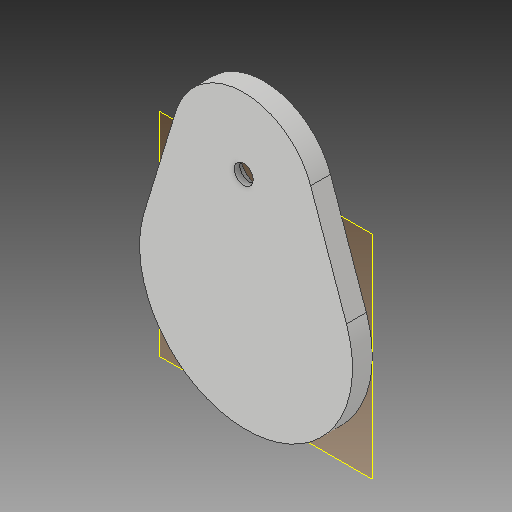
# Autodesk Inventor part: case part 1
Saved by Autodesk Inventor 2017 (Build 210142000, 142)
## iProperties
Created: 2018-04-16
Part Number: case part 1
Material: Generic
Document SubType Name: Modeling
Designer: RKL
Density: 1 g/cm^3
Appearance: Default
Author: RKL
Autodesk Inventor part; units mm, degrees
ref_plane "YZ Plane" through (0, 0, 0) normal (1, 0, 0) x (0, 1, 0)
ref_plane "XZ Plane" through (0, 0, 0) normal (0, 1, 0) x (-1, 0, 0)
ref_plane "XY Plane" through (0, 0, 0) normal (0, 0, 1) x (1, 0, 0)
ref_plane "Work Plane1" through (0, 0, 0) normal (0, 0, 1) x (1, 0, 0)
sketch "Sketch1" plane through (0, 0, 0) normal (0, 0, 1) x (1, 0, 0)
  circle A0 centre (0, 0) radius 17.5 projected
  circle A1 centre (-1.6604, 79.9828) radius 17.5 projected
  circle A2 centre (0, 0) radius 6.7352 construction
  arc A3 (6.3355, 64.3254) -> (5.4562, 67.7807) centre (-13.8587, 61.0262) ccw construction
  arc A4 (5.4562, 67.7807) -> (4.2455, 67.8673) centre (0, 0) ccw construction
  arc A5 (4.2455, 67.8673) -> (2.8834, 64.5723) centre (22.4025, 58.4327) ccw construction
  arc A6 (2.8834, 64.5723) -> (1.7304, 64.6134) centre (0, 0) ccw construction
  arc A7 (1.7304, 64.6134) -> (0.6069, 67.9973) centre (-18.1769, 59.882) ccw construction
  arc A8 (0.6069, 67.9973) -> (-0.6069, 67.9973) centre (0, 0) ccw construction
  arc A9 (-0.6069, 67.9973) -> (-1.7304, 64.6134) centre (18.1769, 59.882) ccw construction
  arc A10 (-1.7304, 64.6134) -> (-2.8834, 64.5723) centre (0, 0) ccw construction
  arc A11 (-2.8834, 64.5723) -> (-4.2455, 67.8673) centre (-22.4025, 58.4327) ccw construction
  arc A12 (-4.2455, 67.8673) -> (-5.4562, 67.7807) centre (0, 0) ccw construction
  arc A13 (-5.4562, 67.7807) -> (-6.3355, 64.3254) centre (13.8587, 61.0262) ccw construction
  arc A14 (-6.3355, 64.3254) -> (-7.4826, 64.202) centre (0, 0) ccw construction
  arc A15 (-7.4826, 64.202) -> (-9.0763, 67.3915) centre (-26.514, 56.6857) ccw construction
  arc A16 (-9.0763, 67.3915) -> (-10.2777, 67.2188) centre (0, 0) ccw construction
  arc A17 (-10.2777, 67.2188) -> (-10.9083, 63.7095) centre (9.4698, 61.8594) ccw construction
  arc A18 (-10.9083, 63.7095) -> (-12.0437, 63.5047) centre (0, 0) ccw construction
  arc A19 (-12.0437, 63.5047) -> (-13.8608, 66.5723) centre (-30.4904, 54.6497) ccw construction
  arc A20 (-13.8608, 66.5723) -> (-15.0469, 66.3143) centre (0, 0) ccw construction
  arc A21 (-15.0469, 66.3143) -> (-15.4255, 62.769) centre (5.0327, 62.3773) ccw construction
  arc A22 (-15.4255, 62.769) -> (-16.5434, 62.4837) centre (0, 0) ccw construction
  arc A23 (-16.5434, 62.4837) -> (-18.5747, 65.4139) centre (-34.3113, 52.3353) ccw construction
  arc A24 (-18.5747, 65.4139) -> (-19.7394, 65.0719) centre (0, 0) ccw construction
  arc A25 (-19.7394, 65.0719) -> (-19.8641, 61.5086) centre (0.5699, 62.5774) ccw construction
  arc A26 (-19.8641, 61.5086) -> (-20.9588, 61.1443) centre (0, 0) ccw construction
  arc A27 (-20.9588, 61.1443) -> (-23.194, 63.9221) centre (-37.9575, 49.7543) ccw construction
  arc A28 (-23.194, 63.9221) -> (-24.3312, 63.498) centre (0, 0) ccw construction
  arc A29 (-24.3312, 63.498) -> (-24.2014, 59.9348) centre (-3.8958, 62.4586) ccw construction
  arc A30 (-24.2014, 59.9348) -> (-25.2673, 59.4933) centre (0, 0) ccw construction
  arc A31 (-25.2673, 59.4933) -> (-27.695, 62.1046) centre (-41.4102, 46.9196) ccw construction
  arc A32 (-27.695, 62.1046) -> (-28.7991, 61.6004) centre (0, 0) ccw construction
  arc A33 (-28.7991, 61.6004) -> (-28.4155, 58.0556) centre (-8.3416, 62.0216) ccw construction
  arc A34 (-28.4155, 58.0556) -> (-29.4472, 57.5392) centre (0, 0) ccw construction
  arc A35 (-29.4472, 57.5392) -> (-32.055, 59.9706) centre (-44.6519, 43.8459) ccw construction
  arc A36 (-32.055, 59.9706) -> (-33.1203, 59.3889) centre (0, 0) ccw construction
  arc A37 (-33.1203, 59.3889) -> (-32.4847, 55.8806) centre (-12.7449, 61.2685) ccw construction
  arc A38 (-32.4847, 55.8806) -> (-33.4769, 55.2918) centre (0, 0) ccw construction
  arc A39 (-33.4769, 55.2918) -> (-36.2516, 57.5311) centre (-47.6661, 40.5488) ccw construction
  arc A40 (-36.2516, 57.5311) -> (-37.2727, 56.8749) centre (0, 0) ccw construction
  arc A41 (-37.2727, 56.8749) -> (-36.3884, 53.4207) centre (-17.0833, 60.2031) ccw construction
  arc A42 (-36.3884, 53.4207) -> (-37.3361, 52.7627) centre (0, 0) ccw construction
  arc A43 (-37.3361, 52.7627) -> (-40.2634, 54.7983) centre (-50.4373, 37.045) ccw construction
  arc A44 (-40.2634, 54.7983) -> (-41.2351, 54.0709) centre (0, 0) ccw construction
  arc A45 (-41.2351, 54.0709) -> (-40.1067, 50.6887) centre (-21.3346, 58.831) ccw construction
  arc A46 (-40.1067, 50.6887) -> (-41.005, 49.9648) centre (0, 0) ccw construction
  arc A47 (-41.005, 49.9648) -> (-44.0701, 51.7864) centre (-52.9516, 33.3525) ccw construction
  arc A48 (-44.0701, 51.7864) -> (-44.9874, 50.9915) centre (0, 0) ccw construction
  arc A49 (-44.9874, 50.9915) -> (-43.6206, 47.6984) centre (-25.4772, 57.1592) ccw construction
  arc A50 (-43.6206, 47.6984) -> (-44.465, 46.9122) centre (0, 0) ccw construction
  arc A51 (-44.465, 46.9122) -> (-47.6522, 48.5105) centre (-55.196, 29.49) ccw construction
  arc A52 (-47.6522, 48.5105) -> (-48.5105, 47.6522) centre (0, 0) ccw construction
  arc A53 (-48.5105, 47.6522) -> (-46.9122, 44.465) centre (-29.49, 55.196) ccw construction
  arc A54 (-46.9122, 44.465) -> (-47.6984, 43.6206) centre (0, 0) ccw construction
  arc A55 (-47.6984, 43.6206) -> (-50.9915, 44.9874) centre (-57.1592, 25.4772) ccw construction
  arc A56 (-50.9915, 44.9874) -> (-51.7864, 44.0701) centre (0, 0) ccw construction
  arc A57 (-51.7864, 44.0701) -> (-49.9648, 41.005) centre (-33.3525, 52.9516) ccw construction
  arc A58 (-49.9648, 41.005) -> (-50.6887, 40.1067) centre (0, 0) ccw construction
  arc A59 (-50.6887, 40.1067) -> (-54.0709, 41.2351) centre (-58.831, 21.3346) ccw construction
  arc A60 (-54.0709, 41.2351) -> (-54.7983, 40.2634) centre (0, 0) ccw construction
  arc A61 (-54.7983, 40.2634) -> (-52.7627, 37.3361) centre (-37.045, 50.4373) ccw construction
  arc A62 (-52.7627, 37.3361) -> (-53.4207, 36.3884) centre (0, 0) ccw construction
  arc A63 (-53.4207, 36.3884) -> (-56.8749, 37.2727) centre (-60.2031, 17.0833) ccw construction
  arc A64 (-56.8749, 37.2727) -> (-57.5311, 36.2516) centre (0, 0) ccw construction
  arc A65 (-57.5311, 36.2516) -> (-55.2918, 33.4769) centre (-40.5488, 47.6661) ccw construction
  arc A66 (-55.2918, 33.4769) -> (-55.8806, 32.4847) centre (0, 0) ccw construction
  arc A67 (-55.8806, 32.4847) -> (-59.3889, 33.1203) centre (-61.2685, 12.7449) ccw construction
  arc A68 (-59.3889, 33.1203) -> (-59.9706, 32.055) centre (0, 0) ccw construction
  arc A69 (-59.9706, 32.055) -> (-57.5392, 29.4472) centre (-43.8459, 44.6519) ccw construction
  arc A70 (-57.5392, 29.4472) -> (-58.0556, 28.4155) centre (0, 0) ccw construction
  arc A71 (-58.0556, 28.4155) -> (-61.6004, 28.7991) centre (-62.0216, 8.3416) ccw construction
  arc A72 (-61.6004, 28.7991) -> (-62.1046, 27.695) centre (0, 0) ccw construction
  arc A73 (-62.1046, 27.695) -> (-59.4933, 25.2673) centre (-46.9196, 41.4102) ccw construction
  arc A74 (-59.4933, 25.2673) -> (-59.9348, 24.2014) centre (0, 0) ccw construction
  arc A75 (-59.9348, 24.2014) -> (-63.498, 24.3312) centre (-62.4586, 3.8958) ccw construction
  arc A76 (-63.498, 24.3312) -> (-63.9221, 23.194) centre (0, 0) ccw construction
  arc A77 (-63.9221, 23.194) -> (-61.1443, 20.9588) centre (-49.7543, 37.9575) ccw construction
  arc A78 (-61.1443, 20.9588) -> (-61.5086, 19.8641) centre (0, 0) ccw construction
  arc A79 (-61.5086, 19.8641) -> (-65.0719, 19.7394) centre (-62.5774, -0.5699) ccw construction
  arc A80 (-65.0719, 19.7394) -> (-65.4139, 18.5747) centre (0, 0) ccw construction
  arc A81 (-65.4139, 18.5747) -> (-62.4837, 16.5434) centre (-52.3353, 34.3113) ccw construction
  arc A82 (-62.4837, 16.5434) -> (-62.769, 15.4255) centre (0, 0) ccw construction
  arc A83 (-62.769, 15.4255) -> (-66.3143, 15.0469) centre (-62.3773, -5.0327) ccw construction
  arc A84 (-66.3143, 15.0469) -> (-66.5723, 13.8608) centre (0, 0) ccw construction
  arc A85 (-66.5723, 13.8608) -> (-63.5047, 12.0437) centre (-54.6497, 30.4904) ccw construction
  arc A86 (-63.5047, 12.0437) -> (-63.7095, 10.9083) centre (0, 0) ccw construction
  arc A87 (-63.7095, 10.9083) -> (-67.2188, 10.2777) centre (-61.8594, -9.4698) ccw construction
  arc A88 (-67.2188, 10.2777) -> (-67.3915, 9.0763) centre (0, 0) ccw construction
  arc A89 (-67.3915, 9.0763) -> (-64.202, 7.4826) centre (-56.6857, 26.514) ccw construction
  arc A90 (-64.202, 7.4826) -> (-64.3254, 6.3355) centre (0, 0) ccw construction
  arc A91 (-64.3254, 6.3355) -> (-67.7807, 5.4562) centre (-61.0262, -13.8587) ccw construction
  arc A92 (-67.7807, 5.4562) -> (-67.8673, 4.2455) centre (0, 0) ccw construction
  arc A93 (-67.8673, 4.2455) -> (-64.5723, 2.8834) centre (-58.4327, 22.4025) ccw construction
  arc A94 (-64.5723, 2.8834) -> (-64.6134, 1.7304) centre (0, 0) ccw construction
  arc A95 (-64.6134, 1.7304) -> (-67.9973, 0.6069) centre (-59.882, -18.1769) ccw construction
  arc A96 (-67.9973, 0.6069) -> (-67.9973, -0.6069) centre (0, 0) ccw construction
  arc A97 (-67.9973, -0.6069) -> (-64.6134, -1.7304) centre (-59.882, 18.1769) ccw construction
  arc A98 (-64.6134, -1.7304) -> (-64.5723, -2.8834) centre (0, 0) ccw construction
  arc A99 (-64.5723, -2.8834) -> (-67.8673, -4.2455) centre (-58.4327, -22.4025) ccw construction
  arc A100 (-67.8673, -4.2455) -> (-67.7807, -5.4562) centre (0, 0) ccw construction
  arc A101 (-67.7807, -5.4562) -> (-64.3254, -6.3355) centre (-61.0262, 13.8587) ccw construction
  arc A102 (-64.3254, -6.3355) -> (-64.202, -7.4826) centre (0, 0) ccw construction
  arc A103 (-64.202, -7.4826) -> (-67.3915, -9.0763) centre (-56.6857, -26.514) ccw construction
  arc A104 (-67.3915, -9.0763) -> (-67.2188, -10.2777) centre (0, 0) ccw construction
  arc A105 (-67.2188, -10.2777) -> (-63.7095, -10.9083) centre (-61.8594, 9.4698) ccw construction
  arc A106 (-63.7095, -10.9083) -> (-63.5047, -12.0437) centre (0, 0) ccw construction
  arc A107 (-63.5047, -12.0437) -> (-66.5723, -13.8608) centre (-54.6497, -30.4904) ccw construction
  arc A108 (-66.5723, -13.8608) -> (-66.3143, -15.0469) centre (0, 0) ccw construction
  arc A109 (-66.3143, -15.0469) -> (-62.769, -15.4255) centre (-62.3773, 5.0327) ccw construction
  arc A110 (-62.769, -15.4255) -> (-62.4837, -16.5434) centre (0, 0) ccw construction
  arc A111 (-62.4837, -16.5434) -> (-65.4139, -18.5747) centre (-52.3353, -34.3113) ccw construction
  arc A112 (-65.4139, -18.5747) -> (-65.0719, -19.7394) centre (0, 0) ccw construction
  arc A113 (-65.0719, -19.7394) -> (-61.5086, -19.8641) centre (-62.5774, 0.5699) ccw construction
  arc A114 (-61.5086, -19.8641) -> (-61.1443, -20.9588) centre (0, 0) ccw construction
  arc A115 (-61.1443, -20.9588) -> (-63.9221, -23.194) centre (-49.7543, -37.9575) ccw construction
  arc A116 (-63.9221, -23.194) -> (-63.498, -24.3312) centre (0, 0) ccw construction
  arc A117 (-63.498, -24.3312) -> (-59.9348, -24.2014) centre (-62.4586, -3.8958) ccw construction
  arc A118 (-59.9348, -24.2014) -> (-59.4933, -25.2673) centre (0, 0) ccw construction
  arc A119 (-59.4933, -25.2673) -> (-62.1046, -27.695) centre (-46.9196, -41.4102) ccw construction
  arc A120 (-62.1046, -27.695) -> (-61.6004, -28.7991) centre (0, 0) ccw construction
  arc A121 (-61.6004, -28.7991) -> (-58.0556, -28.4155) centre (-62.0216, -8.3416) ccw construction
  arc A122 (-58.0556, -28.4155) -> (-57.5392, -29.4472) centre (0, 0) ccw construction
  arc A123 (-57.5392, -29.4472) -> (-59.9706, -32.055) centre (-43.8459, -44.6519) ccw construction
  arc A124 (-59.9706, -32.055) -> (-59.3889, -33.1203) centre (0, 0) ccw construction
  arc A125 (-59.3889, -33.1203) -> (-55.8806, -32.4847) centre (-61.2685, -12.7449) ccw construction
  arc A126 (-55.8806, -32.4847) -> (-55.2918, -33.4769) centre (0, 0) ccw construction
  arc A127 (-55.2918, -33.4769) -> (-57.5311, -36.2516) centre (-40.5488, -47.6661) ccw construction
  arc A128 (-57.5311, -36.2516) -> (-56.8749, -37.2727) centre (0, 0) ccw construction
  arc A129 (-56.8749, -37.2727) -> (-53.4207, -36.3884) centre (-60.2031, -17.0833) ccw construction
  arc A130 (-53.4207, -36.3884) -> (-52.7627, -37.3361) centre (0, 0) ccw construction
  arc A131 (-52.7627, -37.3361) -> (-54.7983, -40.2634) centre (-37.045, -50.4373) ccw construction
  arc A132 (-54.7983, -40.2634) -> (-54.0709, -41.2351) centre (0, 0) ccw construction
  arc A133 (-54.0709, -41.2351) -> (-50.6887, -40.1067) centre (-58.831, -21.3346) ccw construction
  arc A134 (-50.6887, -40.1067) -> (-49.9648, -41.005) centre (0, 0) ccw construction
  arc A135 (-49.9648, -41.005) -> (-51.7864, -44.0701) centre (-33.3525, -52.9516) ccw construction
  arc A136 (-51.7864, -44.0701) -> (-50.9915, -44.9874) centre (0, 0) ccw construction
  arc A137 (-50.9915, -44.9874) -> (-47.6984, -43.6206) centre (-57.1592, -25.4772) ccw construction
  arc A138 (-47.6984, -43.6206) -> (-46.9122, -44.465) centre (0, 0) ccw construction
  arc A139 (-46.9122, -44.465) -> (-48.5105, -47.6522) centre (-29.49, -55.196) ccw construction
  arc A140 (-48.5105, -47.6522) -> (-47.6522, -48.5105) centre (0, 0) ccw construction
  arc A141 (-47.6522, -48.5105) -> (-44.465, -46.9122) centre (-55.196, -29.49) ccw construction
  arc A142 (-44.465, -46.9122) -> (-43.6206, -47.6984) centre (0, 0) ccw construction
  arc A143 (-43.6206, -47.6984) -> (-44.9874, -50.9915) centre (-25.4772, -57.1592) ccw construction
  arc A144 (-44.9874, -50.9915) -> (-44.0701, -51.7864) centre (0, 0) ccw construction
  arc A145 (-44.0701, -51.7864) -> (-41.005, -49.9648) centre (-52.9516, -33.3525) ccw construction
  arc A146 (-41.005, -49.9648) -> (-40.1067, -50.6887) centre (0, 0) ccw construction
  arc A147 (-40.1067, -50.6887) -> (-41.2351, -54.0709) centre (-21.3346, -58.831) ccw construction
  arc A148 (-41.2351, -54.0709) -> (-40.2634, -54.7983) centre (0, 0) ccw construction
  arc A149 (-40.2634, -54.7983) -> (-37.3361, -52.7627) centre (-50.4373, -37.045) ccw construction
  arc A150 (-37.3361, -52.7627) -> (-36.3884, -53.4207) centre (0, 0) ccw construction
  arc A151 (-36.3884, -53.4207) -> (-37.2727, -56.8749) centre (-17.0833, -60.2031) ccw construction
  arc A152 (-37.2727, -56.8749) -> (-36.2516, -57.5311) centre (0, 0) ccw construction
  arc A153 (-36.2516, -57.5311) -> (-33.4769, -55.2918) centre (-47.6661, -40.5488) ccw construction
  arc A154 (-33.4769, -55.2918) -> (-32.4847, -55.8806) centre (0, 0) ccw construction
  arc A155 (-32.4847, -55.8806) -> (-33.1203, -59.3889) centre (-12.7449, -61.2685) ccw construction
  arc A156 (-33.1203, -59.3889) -> (-32.055, -59.9706) centre (0, 0) ccw construction
  arc A157 (-32.055, -59.9706) -> (-29.4472, -57.5392) centre (-44.6519, -43.8459) ccw construction
  arc A158 (-29.4472, -57.5392) -> (-28.4155, -58.0556) centre (0, 0) ccw construction
  arc A159 (-28.4155, -58.0556) -> (-28.7991, -61.6004) centre (-8.3416, -62.0216) ccw construction
  arc A160 (-28.7991, -61.6004) -> (-27.695, -62.1046) centre (0, 0) ccw construction
  arc A161 (-27.695, -62.1046) -> (-25.2673, -59.4933) centre (-41.4102, -46.9196) ccw construction
  arc A162 (-25.2673, -59.4933) -> (-24.2014, -59.9348) centre (0, 0) ccw construction
  arc A163 (-24.2014, -59.9348) -> (-24.3312, -63.498) centre (-3.8958, -62.4586) ccw construction
  arc A164 (-24.3312, -63.498) -> (-23.194, -63.9221) centre (0, 0) ccw construction
  arc A165 (-23.194, -63.9221) -> (-20.9588, -61.1443) centre (-37.9575, -49.7543) ccw construction
  arc A166 (-20.9588, -61.1443) -> (-19.8641, -61.5086) centre (0, 0) ccw construction
  arc A167 (-19.8641, -61.5086) -> (-19.7394, -65.0719) centre (0.5699, -62.5774) ccw construction
  arc A168 (-19.7394, -65.0719) -> (-18.5747, -65.4139) centre (0, 0) ccw construction
  arc A169 (-18.5747, -65.4139) -> (-16.5434, -62.4837) centre (-34.3113, -52.3353) ccw construction
  arc A170 (-16.5434, -62.4837) -> (-15.4255, -62.769) centre (0, 0) ccw construction
  arc A171 (-15.4255, -62.769) -> (-15.0469, -66.3143) centre (5.0327, -62.3773) ccw construction
  arc A172 (-15.0469, -66.3143) -> (-13.8608, -66.5723) centre (0, 0) ccw construction
  arc A173 (-13.8608, -66.5723) -> (-12.0437, -63.5047) centre (-30.4904, -54.6497) ccw construction
  arc A174 (-12.0437, -63.5047) -> (-10.9083, -63.7095) centre (0, 0) ccw construction
  arc A175 (-10.9083, -63.7095) -> (-10.2777, -67.2188) centre (9.4698, -61.8594) ccw construction
  arc A176 (-10.2777, -67.2188) -> (-9.0763, -67.3915) centre (0, 0) ccw construction
  arc A177 (-9.0763, -67.3915) -> (-7.4826, -64.202) centre (-26.514, -56.6857) ccw construction
  arc A178 (-7.4826, -64.202) -> (-6.3355, -64.3254) centre (0, 0) ccw construction
  arc A179 (-6.3355, -64.3254) -> (-5.4562, -67.7807) centre (13.8587, -61.0262) ccw construction
  arc A180 (-5.4562, -67.7807) -> (-4.2455, -67.8673) centre (0, 0) ccw construction
  arc A181 (-4.2455, -67.8673) -> (-2.8834, -64.5723) centre (-22.4025, -58.4327) ccw construction
  arc A182 (-2.8834, -64.5723) -> (-1.7304, -64.6134) centre (0, 0) ccw construction
  arc A183 (-1.7304, -64.6134) -> (-0.6069, -67.9973) centre (18.1769, -59.882) ccw construction
  arc A184 (-0.6069, -67.9973) -> (0.6069, -67.9973) centre (0, 0) ccw construction
  arc A185 (0.6069, -67.9973) -> (1.7304, -64.6134) centre (-18.1769, -59.882) ccw construction
  arc A186 (1.7304, -64.6134) -> (2.8834, -64.5723) centre (0, 0) ccw construction
  arc A187 (2.8834, -64.5723) -> (4.2455, -67.8673) centre (22.4025, -58.4327) ccw construction
  arc A188 (4.2455, -67.8673) -> (5.4562, -67.7807) centre (0, 0) ccw construction
  arc A189 (5.4562, -67.7807) -> (6.3355, -64.3254) centre (-13.8587, -61.0262) ccw construction
  arc A190 (6.3355, -64.3254) -> (7.4826, -64.202) centre (0, 0) ccw construction
  arc A191 (7.4826, -64.202) -> (9.0763, -67.3915) centre (26.514, -56.6857) ccw construction
  arc A192 (9.0763, -67.3915) -> (10.2777, -67.2188) centre (0, 0) ccw construction
  arc A193 (10.2777, -67.2188) -> (10.9083, -63.7095) centre (-9.4698, -61.8594) ccw construction
  arc A194 (10.9083, -63.7095) -> (12.0437, -63.5047) centre (0, 0) ccw construction
  arc A195 (12.0437, -63.5047) -> (13.8608, -66.5723) centre (30.4904, -54.6497) ccw construction
  arc A196 (13.8608, -66.5723) -> (15.0469, -66.3143) centre (0, 0) ccw construction
  arc A197 (15.0469, -66.3143) -> (15.4255, -62.769) centre (-5.0327, -62.3773) ccw construction
  arc A198 (15.4255, -62.769) -> (16.5434, -62.4837) centre (0, 0) ccw construction
  arc A199 (16.5434, -62.4837) -> (18.5747, -65.4139) centre (34.3113, -52.3353) ccw construction
  arc A200 (18.5747, -65.4139) -> (19.7394, -65.0719) centre (0, 0) ccw construction
  arc A201 (19.7394, -65.0719) -> (19.8641, -61.5086) centre (-0.5699, -62.5774) ccw construction
  arc A202 (19.8641, -61.5086) -> (20.9588, -61.1443) centre (0, 0) ccw construction
  arc A203 (20.9588, -61.1443) -> (23.194, -63.9221) centre (37.9575, -49.7543) ccw construction
  arc A204 (23.194, -63.9221) -> (24.3312, -63.498) centre (0, 0) ccw construction
  arc A205 (24.3312, -63.498) -> (24.2014, -59.9348) centre (3.8958, -62.4586) ccw construction
  arc A206 (24.2014, -59.9348) -> (25.2673, -59.4933) centre (0, 0) ccw construction
  arc A207 (25.2673, -59.4933) -> (27.695, -62.1046) centre (41.4102, -46.9196) ccw construction
  arc A208 (27.695, -62.1046) -> (28.7991, -61.6004) centre (0, 0) ccw construction
  arc A209 (28.7991, -61.6004) -> (28.4155, -58.0556) centre (8.3416, -62.0216) ccw construction
  arc A210 (28.4155, -58.0556) -> (29.4472, -57.5392) centre (0, 0) ccw construction
  arc A211 (29.4472, -57.5392) -> (32.055, -59.9706) centre (44.6519, -43.8459) ccw construction
  arc A212 (32.055, -59.9706) -> (33.1203, -59.3889) centre (0, 0) ccw construction
  arc A213 (33.1203, -59.3889) -> (32.4847, -55.8806) centre (12.7449, -61.2685) ccw construction
  arc A214 (32.4847, -55.8806) -> (33.4769, -55.2918) centre (0, 0) ccw construction
  arc A215 (33.4769, -55.2918) -> (36.2516, -57.5311) centre (47.6661, -40.5488) ccw construction
  arc A216 (36.2516, -57.5311) -> (37.2727, -56.8749) centre (0, 0) ccw construction
  arc A217 (37.2727, -56.8749) -> (36.3884, -53.4207) centre (17.0833, -60.2031) ccw construction
  arc A218 (36.3884, -53.4207) -> (37.3361, -52.7627) centre (0, 0) ccw construction
  arc A219 (37.3361, -52.7627) -> (40.2634, -54.7983) centre (50.4373, -37.045) ccw construction
  arc A220 (40.2634, -54.7983) -> (41.2351, -54.0709) centre (0, 0) ccw construction
  arc A221 (41.2351, -54.0709) -> (40.1067, -50.6887) centre (21.3346, -58.831) ccw construction
  arc A222 (40.1067, -50.6887) -> (41.005, -49.9648) centre (0, 0) ccw construction
  arc A223 (41.005, -49.9648) -> (44.0701, -51.7864) centre (52.9516, -33.3525) ccw construction
  arc A224 (44.0701, -51.7864) -> (44.9874, -50.9915) centre (0, 0) ccw construction
  arc A225 (44.9874, -50.9915) -> (43.6206, -47.6984) centre (25.4772, -57.1592) ccw construction
  arc A226 (43.6206, -47.6984) -> (44.465, -46.9122) centre (0, 0) ccw construction
  arc A227 (44.465, -46.9122) -> (47.6522, -48.5105) centre (55.196, -29.49) ccw construction
  arc A228 (47.6522, -48.5105) -> (48.5105, -47.6522) centre (0, 0) ccw construction
  arc A229 (48.5105, -47.6522) -> (46.9122, -44.465) centre (29.49, -55.196) ccw construction
  arc A230 (46.9122, -44.465) -> (47.6984, -43.6206) centre (0, 0) ccw construction
  arc A231 (47.6984, -43.6206) -> (50.9915, -44.9874) centre (57.1592, -25.4772) ccw construction
  arc A232 (50.9915, -44.9874) -> (51.7864, -44.0701) centre (0, 0) ccw construction
  arc A233 (51.7864, -44.0701) -> (49.9648, -41.005) centre (33.3525, -52.9516) ccw construction
  arc A234 (49.9648, -41.005) -> (50.6887, -40.1067) centre (0, 0) ccw construction
  arc A235 (50.6887, -40.1067) -> (54.0709, -41.2351) centre (58.831, -21.3346) ccw construction
  arc A236 (54.0709, -41.2351) -> (54.7983, -40.2634) centre (0, 0) ccw construction
  arc A237 (54.7983, -40.2634) -> (52.7627, -37.3361) centre (37.045, -50.4373) ccw construction
  arc A238 (52.7627, -37.3361) -> (53.4207, -36.3884) centre (0, 0) ccw construction
  arc A239 (53.4207, -36.3884) -> (56.8749, -37.2727) centre (60.2031, -17.0833) ccw construction
  arc A240 (56.8749, -37.2727) -> (57.5311, -36.2516) centre (0, 0) ccw construction
  arc A241 (57.5311, -36.2516) -> (55.2918, -33.4769) centre (40.5488, -47.6661) ccw construction
  arc A242 (55.2918, -33.4769) -> (55.8806, -32.4847) centre (0, 0) ccw construction
  arc A243 (55.8806, -32.4847) -> (59.3889, -33.1203) centre (61.2685, -12.7449) ccw construction
  arc A244 (59.3889, -33.1203) -> (59.9706, -32.055) centre (0, 0) ccw construction
  arc A245 (59.9706, -32.055) -> (57.5392, -29.4472) centre (43.8459, -44.6519) ccw construction
  arc A246 (57.5392, -29.4472) -> (58.0556, -28.4155) centre (0, 0) ccw construction
  arc A247 (58.0556, -28.4155) -> (61.6004, -28.7991) centre (62.0216, -8.3416) ccw construction
  arc A248 (61.6004, -28.7991) -> (62.1046, -27.695) centre (0, 0) ccw construction
  arc A249 (62.1046, -27.695) -> (59.4933, -25.2673) centre (46.9196, -41.4102) ccw construction
  arc A250 (59.4933, -25.2673) -> (59.9348, -24.2014) centre (0, 0) ccw construction
  arc A251 (59.9348, -24.2014) -> (63.498, -24.3312) centre (62.4586, -3.8958) ccw construction
  arc A252 (63.498, -24.3312) -> (63.9221, -23.194) centre (0, 0) ccw construction
  arc A253 (63.9221, -23.194) -> (61.1443, -20.9588) centre (49.7543, -37.9575) ccw construction
  arc A254 (61.1443, -20.9588) -> (61.5086, -19.8641) centre (0, 0) ccw construction
  arc A255 (61.5086, -19.8641) -> (65.0719, -19.7394) centre (62.5774, 0.5699) ccw construction
  arc A256 (65.0719, -19.7394) -> (65.4139, -18.5747) centre (0, 0) ccw construction
  arc A257 (65.4139, -18.5747) -> (62.4837, -16.5434) centre (52.3353, -34.3113) ccw construction
  arc A258 (62.4837, -16.5434) -> (62.769, -15.4255) centre (0, 0) ccw construction
  arc A259 (62.769, -15.4255) -> (66.3143, -15.0469) centre (62.3773, 5.0327) ccw construction
  arc A260 (66.3143, -15.0469) -> (66.5723, -13.8608) centre (0, 0) ccw construction
  arc A261 (66.5723, -13.8608) -> (63.5047, -12.0437) centre (54.6497, -30.4904) ccw construction
  arc A262 (63.5047, -12.0437) -> (63.7095, -10.9083) centre (0, 0) ccw construction
  arc A263 (63.7095, -10.9083) -> (67.2188, -10.2777) centre (61.8594, 9.4698) ccw construction
  arc A264 (67.2188, -10.2777) -> (67.3915, -9.0763) centre (0, 0) ccw construction
  arc A265 (67.3915, -9.0763) -> (64.202, -7.4826) centre (56.6857, -26.514) ccw construction
  arc A266 (64.202, -7.4826) -> (64.3254, -6.3355) centre (0, 0) ccw construction
  arc A267 (64.3254, -6.3355) -> (67.7807, -5.4562) centre (61.0262, 13.8587) ccw construction
  arc A268 (67.7807, -5.4562) -> (67.8673, -4.2455) centre (0, 0) ccw construction
  arc A269 (67.8673, -4.2455) -> (64.5723, -2.8834) centre (58.4327, -22.4025) ccw construction
  arc A270 (64.5723, -2.8834) -> (64.6134, -1.7304) centre (0, 0) ccw construction
  arc A271 (64.6134, -1.7304) -> (67.9973, -0.6069) centre (59.882, 18.1769) ccw construction
  arc A272 (67.9973, -0.6069) -> (67.9973, 0.6069) centre (0, 0) ccw construction
  arc A273 (67.9973, 0.6069) -> (64.6134, 1.7304) centre (59.882, -18.1769) ccw construction
  arc A274 (64.6134, 1.7304) -> (64.5723, 2.8834) centre (0, 0) ccw construction
  arc A275 (64.5723, 2.8834) -> (67.8673, 4.2455) centre (58.4327, 22.4025) ccw construction
  arc A276 (67.8673, 4.2455) -> (67.7807, 5.4562) centre (0, 0) ccw construction
  arc A277 (67.7807, 5.4562) -> (64.3254, 6.3355) centre (61.0262, -13.8587) ccw construction
  arc A278 (64.3254, 6.3355) -> (64.202, 7.4826) centre (0, 0) ccw construction
  arc A279 (64.202, 7.4826) -> (67.3915, 9.0763) centre (56.6857, 26.514) ccw construction
  arc A280 (67.3915, 9.0763) -> (67.2188, 10.2777) centre (0, 0) ccw construction
  arc A281 (67.2188, 10.2777) -> (63.7095, 10.9083) centre (61.8594, -9.4698) ccw construction
  arc A282 (63.7095, 10.9083) -> (63.5047, 12.0437) centre (0, 0) ccw construction
  arc A283 (63.5047, 12.0437) -> (66.5723, 13.8608) centre (54.6497, 30.4904) ccw construction
  arc A284 (66.5723, 13.8608) -> (66.3143, 15.0469) centre (0, 0) ccw construction
  arc A285 (66.3143, 15.0469) -> (62.769, 15.4255) centre (62.3773, -5.0327) ccw construction
  arc A286 (62.769, 15.4255) -> (62.4837, 16.5434) centre (0, 0) ccw construction
  arc A287 (62.4837, 16.5434) -> (65.4139, 18.5747) centre (52.3353, 34.3113) ccw construction
  arc A288 (65.4139, 18.5747) -> (65.0719, 19.7394) centre (0, 0) ccw construction
  arc A289 (65.0719, 19.7394) -> (61.5086, 19.8641) centre (62.5774, -0.5699) ccw construction
  arc A290 (61.5086, 19.8641) -> (61.1443, 20.9588) centre (0, 0) ccw construction
  arc A291 (61.1443, 20.9588) -> (63.9221, 23.194) centre (49.7543, 37.9575) ccw construction
  arc A292 (63.9221, 23.194) -> (63.498, 24.3312) centre (0, 0) ccw construction
  arc A293 (63.498, 24.3312) -> (59.9348, 24.2014) centre (62.4586, 3.8958) ccw construction
  arc A294 (59.9348, 24.2014) -> (59.4933, 25.2673) centre (0, 0) ccw construction
  arc A295 (59.4933, 25.2673) -> (62.1046, 27.695) centre (46.9196, 41.4102) ccw construction
  arc A296 (62.1046, 27.695) -> (61.6004, 28.7991) centre (0, 0) ccw construction
  arc A297 (61.6004, 28.7991) -> (58.0556, 28.4155) centre (62.0216, 8.3416) ccw construction
  arc A298 (58.0556, 28.4155) -> (57.5392, 29.4472) centre (0, 0) ccw construction
  arc A299 (57.5392, 29.4472) -> (59.9706, 32.055) centre (43.8459, 44.6519) ccw construction
  arc A300 (59.9706, 32.055) -> (59.3889, 33.1203) centre (0, 0) ccw construction
  arc A301 (59.3889, 33.1203) -> (55.8806, 32.4847) centre (61.2685, 12.7449) ccw construction
  arc A302 (55.8806, 32.4847) -> (55.2918, 33.4769) centre (0, 0) ccw construction
  arc A303 (55.2918, 33.4769) -> (57.5311, 36.2516) centre (40.5488, 47.6661) ccw construction
  arc A304 (57.5311, 36.2516) -> (56.8749, 37.2727) centre (0, 0) ccw construction
  arc A305 (56.8749, 37.2727) -> (53.4207, 36.3884) centre (60.2031, 17.0833) ccw construction
  arc A306 (53.4207, 36.3884) -> (52.7627, 37.3361) centre (0, 0) ccw construction
  arc A307 (52.7627, 37.3361) -> (54.7983, 40.2634) centre (37.045, 50.4373) ccw construction
  arc A308 (54.7983, 40.2634) -> (54.0709, 41.2351) centre (0, 0) ccw construction
  arc A309 (54.0709, 41.2351) -> (50.6887, 40.1067) centre (58.831, 21.3346) ccw construction
  arc A310 (50.6887, 40.1067) -> (49.9648, 41.005) centre (0, 0) ccw construction
  arc A311 (49.9648, 41.005) -> (51.7864, 44.0701) centre (33.3525, 52.9516) ccw construction
  arc A312 (51.7864, 44.0701) -> (50.9915, 44.9874) centre (0, 0) ccw construction
  arc A313 (50.9915, 44.9874) -> (47.6984, 43.6206) centre (57.1592, 25.4772) ccw construction
  arc A314 (47.6984, 43.6206) -> (46.9122, 44.465) centre (0, 0) ccw construction
  arc A315 (46.9122, 44.465) -> (48.5105, 47.6522) centre (29.49, 55.196) ccw construction
  arc A316 (48.5105, 47.6522) -> (47.6522, 48.5105) centre (0, 0) ccw construction
  arc A317 (47.6522, 48.5105) -> (44.465, 46.9122) centre (55.196, 29.49) ccw construction
  arc A318 (44.465, 46.9122) -> (43.6206, 47.6984) centre (0, 0) ccw construction
  arc A319 (43.6206, 47.6984) -> (44.9874, 50.9915) centre (25.4772, 57.1592) ccw construction
  arc A320 (44.9874, 50.9915) -> (44.0701, 51.7864) centre (0, 0) ccw construction
  arc A321 (44.0701, 51.7864) -> (41.005, 49.9648) centre (52.9516, 33.3525) ccw construction
  arc A322 (41.005, 49.9648) -> (40.1067, 50.6887) centre (0, 0) ccw construction
  arc A323 (40.1067, 50.6887) -> (41.2351, 54.0709) centre (21.3346, 58.831) ccw construction
  arc A324 (41.2351, 54.0709) -> (40.2634, 54.7983) centre (0, 0) ccw construction
  arc A325 (40.2634, 54.7983) -> (37.3361, 52.7627) centre (50.4373, 37.045) ccw construction
  arc A326 (37.3361, 52.7627) -> (36.3884, 53.4207) centre (0, 0) ccw construction
  arc A327 (36.3884, 53.4207) -> (37.2727, 56.8749) centre (17.0833, 60.2031) ccw construction
  arc A328 (37.2727, 56.8749) -> (36.2516, 57.5311) centre (0, 0) ccw construction
  arc A329 (36.2516, 57.5311) -> (33.4769, 55.2918) centre (47.6661, 40.5488) ccw construction
  arc A330 (33.4769, 55.2918) -> (32.4847, 55.8806) centre (0, 0) ccw construction
  arc A331 (32.4847, 55.8806) -> (33.1203, 59.3889) centre (12.7449, 61.2685) ccw construction
  arc A332 (33.1203, 59.3889) -> (32.055, 59.9706) centre (0, 0) ccw construction
  arc A333 (32.055, 59.9706) -> (29.4472, 57.5392) centre (44.6519, 43.8459) ccw construction
  arc A334 (29.4472, 57.5392) -> (28.4155, 58.0556) centre (0, 0) ccw construction
  arc A335 (28.4155, 58.0556) -> (28.7991, 61.6004) centre (8.3416, 62.0216) ccw construction
  arc A336 (28.7991, 61.6004) -> (27.695, 62.1046) centre (0, 0) ccw construction
  arc A337 (27.695, 62.1046) -> (25.2673, 59.4933) centre (41.4102, 46.9196) ccw construction
  arc A338 (25.2673, 59.4933) -> (24.2014, 59.9348) centre (0, 0) ccw construction
  arc A339 (24.2014, 59.9348) -> (24.3312, 63.498) centre (3.8958, 62.4586) ccw construction
  arc A340 (24.3312, 63.498) -> (23.194, 63.9221) centre (0, 0) ccw construction
  arc A341 (23.194, 63.9221) -> (20.9588, 61.1443) centre (37.9575, 49.7543) ccw construction
  arc A342 (20.9588, 61.1443) -> (19.8641, 61.5086) centre (0, 0) ccw construction
  arc A343 (19.8641, 61.5086) -> (19.7394, 65.0719) centre (-0.5699, 62.5774) ccw construction
  arc A344 (19.7394, 65.0719) -> (18.5747, 65.4139) centre (0, 0) ccw construction
  arc A345 (18.5747, 65.4139) -> (16.5434, 62.4837) centre (34.3113, 52.3353) ccw construction
  arc A346 (16.5434, 62.4837) -> (15.4255, 62.769) centre (0, 0) ccw construction
  arc A347 (15.4255, 62.769) -> (15.0469, 66.3143) centre (-5.0327, 62.3773) ccw construction
  arc A348 (15.0469, 66.3143) -> (13.8608, 66.5723) centre (0, 0) ccw construction
  arc A349 (13.8608, 66.5723) -> (12.0437, 63.5047) centre (30.4904, 54.6497) ccw construction
  arc A350 (12.0437, 63.5047) -> (10.9083, 63.7095) centre (0, 0) ccw construction
  arc A351 (10.9083, 63.7095) -> (10.2777, 67.2188) centre (-9.4698, 61.8594) ccw construction
  arc A352 (10.2777, 67.2188) -> (9.0763, 67.3915) centre (0, 0) ccw construction
  arc A353 (9.0763, 67.3915) -> (7.4826, 64.202) centre (26.514, 56.6857) ccw construction
  arc A354 (7.4826, 64.202) -> (6.3355, 64.3254) centre (0, 0) ccw construction
  line L0 (1.5013, 85.9298) -> (4.2866, 76.8211) construction
  line L1 (4.2866, 76.8211) -> (-4.822, 74.0358) construction
  line L2 (-4.822, 74.0358) -> (-7.6074, 83.1444) construction
  line L3 (-7.6074, 83.1444) -> (1.5013, 85.9298) construction
  arc A355 (-2.5253, 42.7312) -> (-0.1223, 36.0097) centre (25.3334, 48.9006) ccw construction
  arc A356 (-0.1223, 36.0097) -> (2.4319, 36.1735) centre (-1.6604, 79.9828) ccw construction
  arc A357 (2.4319, 36.1735) -> (3.9565, 43.1469) centre (-24.462, 45.7067) ccw construction
  arc A358 (3.9565, 43.1469) -> (6.0888, 43.5359) centre (-1.6604, 79.9828) ccw construction
  arc A359 (6.0888, 43.5359) -> (9.9772, 37.5497) centre (31.7738, 55.9636) ccw construction
  arc A360 (9.9772, 37.5497) -> (12.4247, 38.2981) centre (-1.6604, 79.9828) ccw construction
  arc A361 (12.4247, 38.2981) -> (12.3001, 45.4352) centre (-15.9428, 41.3722) ccw construction
  arc A362 (12.3001, 45.4352) -> (14.2852, 46.3054) centre (-1.6604, 79.9828) ccw construction
  arc A363 (14.2852, 46.3054) -> (19.4492, 41.3773) centre (36.4118, 64.3215) ccw construction
  arc A364 (19.4492, 41.3773) -> (21.6582, 42.67) centre (-1.6604, 79.9828) ccw construction
  arc A365 (21.6582, 42.67) -> (19.891, 49.5859) centre (-6.6536, 39.1192) ccw construction
  arc A366 (19.891, 49.5859) -> (21.6219, 50.8905) centre (-1.6604, 79.9828) ccw construction
  arc A367 (21.6219, 50.8905) -> (27.7833, 47.2861) centre (38.9973, 73.5237) ccw construction
  arc A368 (27.7833, 47.2861) -> (29.6346, 49.0534) centre (-1.6604, 79.9828) ccw construction
  arc A369 (29.6346, 49.0534) -> (26.32, 55.3754) centre (2.9048, 39.0691) ccw construction
  arc A370 (26.32, 55.3754) -> (27.7035, 57.0439) centre (-1.6604, 79.9828) ccw construction
  arc A371 (27.7035, 57.0439) -> (34.53, 54.9576) centre (39.3909, 83.0741) ccw construction
  arc A372 (34.53, 54.9576) -> (35.9238, 57.1042) centre (-1.6604, 79.9828) ccw construction
  arc A373 (35.9238, 57.1042) -> (31.2407, 62.4914) centre (12.2171, 41.2248) ccw construction
  arc A374 (31.2407, 62.4914) -> (32.2021, 64.434) centre (-1.6604, 79.9828) ccw construction
  arc A375 (32.2021, 64.434) -> (39.3257, 63.9782) centre (37.5715, 92.4579) ccw construction
  arc A376 (39.3257, 63.9782) -> (40.1869, 66.3884) centre (-1.6604, 79.9828) ccw construction
  arc A377 (40.1869, 66.3884) -> (34.3876, 70.5504) centre (20.7812, 45.4698) ccw construction
  arc A378 (34.3876, 70.5504) -> (34.8751, 72.6623) centre (-1.6604, 79.9828) ccw construction
  arc A379 (34.8751, 72.6623) -> (41.9118, 73.8617) centre (33.637, 101.1691) ccw construction
  arc A380 (41.9118, 73.8617) -> (42.194, 76.4055) centre (-1.6604, 79.9828) ccw construction
  arc A381 (42.194, 76.4055) -> (35.5912, 79.1179) centre (28.1355, 51.5755) ccw construction
  arc A382 (35.5912, 79.1179) -> (35.5785, 81.2853) centre (-1.6604, 79.9828) ccw construction
  arc A383 (35.5785, 81.2853) -> (42.1489, 84.0751) centre (27.7997, 108.7382) ccw construction
  arc A384 (42.1489, 84.0751) -> (41.8368, 86.6154) centre (-1.6604, 79.9828) ccw construction
  arc A385 (41.8368, 86.6154) -> (34.7865, 87.732) centre (33.8835, 59.2126) ccw construction
  arc A386 (34.7865, 87.732) -> (34.2743, 89.8381) centre (-1.6604, 79.9828) ccw construction
  arc A387 (34.2743, 89.8381) -> (40.0243, 94.0679) centre (20.3741, 114.757) ccw construction
  arc A388 (40.0243, 94.0679) -> (39.1348, 96.4678) centre (-1.6604, 79.9828) ccw construction
  arc A389 (39.1348, 96.4678) -> (32.017, 95.9283) centre (37.7154, 67.9695) ccw construction
  arc A390 (32.017, 95.9283) -> (31.0329, 97.8595) centre (-1.6604, 79.9828) ccw construction
  arc A391 (31.0329, 97.8595) -> (35.6524, 103.3014) centre (11.7607, 118.9012) ccw construction
  arc A392 (35.6524, 103.3014) -> (34.2334, 105.4314) centre (-1.6604, 79.9828) ccw construction
  arc A393 (34.2334, 105.4314) -> (27.4319, 103.2651) centre (39.4244, 77.374) ccw construction
  arc A394 (27.4319, 103.2651) -> (26.029, 104.9172) centre (-1.6604, 79.9828) ccw construction
  arc A395 (26.029, 104.9172) -> (29.269, 111.2777) centre (2.4237, 120.9472) ccw construction
  arc A396 (29.269, 111.2777) -> (27.397, 113.0232) centre (-1.6604, 79.9828) ccw construction
  arc A397 (27.397, 113.0232) -> (21.2785, 109.3466) centre (38.9186, 86.9191) ccw construction
  arc A398 (21.2785, 109.3466) -> (19.5323, 110.6307) centre (-1.6604, 79.9828) ccw construction
  arc A399 (19.5323, 110.6307) -> (21.2182, 117.567) centre (-7.1334, 120.7849) ccw construction
  arc A400 (21.2182, 117.567) -> (18.9942, 118.8336) centre (-1.6604, 79.9828) ccw construction
  arc A401 (18.9942, 118.8336) -> (13.8884, 113.8452) centre (36.2252, 96.0903) ccw construction
  arc A402 (13.8884, 113.8452) -> (11.8932, 114.692) centre (-1.6604, 79.9828) ccw construction
  arc A403 (11.8932, 114.692) -> (11.934, 121.83) centre (-16.3955, 118.4229) ccw construction
  arc A404 (11.934, 121.83) -> (9.4778, 122.5497) centre (-1.6604, 79.9828) ccw construction
  arc A405 (9.4778, 122.5497) -> (5.6601, 116.5182) centre (31.4893, 104.3931) ccw construction
  arc A406 (5.6601, 116.5182) -> (3.5233, 116.8821) centre (-1.6604, 79.9828) ccw construction
  arc A407 (3.5233, 116.8821) -> (1.9169, 123.8371) centre (-24.8632, 113.9886) ccw construction
  arc A408 (1.9169, 123.8371) -> (-0.6391, 123.9709) centre (-1.6604, 79.9828) ccw construction
  arc A409 (-0.6391, 123.9709) -> (-2.9629, 117.2216) centre (24.9663, 111.38) ccw construction
  arc A410 (-2.9629, 117.2216) -> (-5.126, 117.0829) centre (-1.6604, 79.9828) ccw construction
  arc A411 (-5.126, 117.0829) -> (-8.293, 123.48) centre (-32.0801, 107.721) ccw construction
  arc A412 (-8.293, 123.48) -> (-10.811, 123.0207) centre (-1.6604, 79.9828) ccw construction
  arc A413 (-10.811, 123.0207) -> (-11.5157, 115.9174) centre (17.0079, 116.6742) ccw construction
  arc A414 (-11.5157, 115.9174) -> (-13.5884, 115.2836) centre (-1.6604, 79.9828) ccw construction
  arc A415 (-13.5884, 115.2836) -> (-18.1454, 120.7779) centre (-37.657, 99.958) ccw construction
  arc A416 (-18.1454, 120.7779) -> (-20.4895, 119.7504) centre (-1.6604, 79.9828) ccw construction
  arc A417 (-20.4895, 119.7504) -> (-19.5371, 112.676) centre (8.0431, 119.9904) ccw construction
  arc A418 (-19.5371, 112.676) -> (-21.4078, 111.5813) centre (-1.6604, 79.9828) ccw construction
  arc A419 (-21.4078, 111.5813) -> (-27.1091, 115.8766) centre (-41.2933, 91.1182) ccw construction
  arc A420 (-27.1091, 115.8766) -> (-29.153, 114.3361) centre (-1.6604, 79.9828) ccw construction
  arc A421 (-29.153, 114.3361) -> (-26.5948, 107.6721) centre (-1.4449, 121.1497) ccw construction
  arc A422 (-26.5948, 107.6721) -> (-28.1627, 106.1755) centre (-1.6604, 79.9828) ccw construction
  arc A423 (-28.1627, 106.1755) -> (-34.7008, 109.0402) centre (-42.793, 81.6781) ccw construction
  arc A424 (-34.7008, 109.0402) -> (-36.3344, 107.0699) centre (-1.6604, 79.9828) ccw construction
  arc A425 (-36.3344, 107.0699) -> (-32.3083, 101.1755) centre (-10.9444, 120.0898) ccw construction
  arc A426 (-32.3083, 101.1755) -> (-33.4887, 99.3576) centre (-1.6604, 79.9828) ccw construction
  arc A427 (-33.4887, 99.3576) -> (-40.5112, 100.6373) centre (-42.0752, 72.1465) ccw construction
  arc A428 (-40.5112, 100.6373) -> (-41.6465, 98.3434) centre (-1.6604, 79.9828) ccw construction
  arc A429 (-41.6465, 98.3434) -> (-36.3696, 93.5363) centre (-19.9435, 116.8676) ccw construction
  arc A430 (-36.3696, 93.5363) -> (-37.0989, 91.4952) centre (-1.6604, 79.9828) ccw construction
  arc A431 (-37.0989, 91.4952) -> (-44.2273, 91.1209) centre (-39.1787, 63.0375) ccw construction
  arc A432 (-44.2273, 91.1209) -> (-44.8029, 88.627) centre (-1.6604, 79.9828) ccw construction
  arc A433 (-44.8029, 88.627) -> (-38.5597, 85.1665) centre (-27.9569, 111.657) ccw construction
  arc A434 (-38.5597, 85.1665) -> (-38.7986, 83.0122) centre (-1.6604, 79.9828) ccw construction
  arc A435 (-38.7986, 83.0122) -> (-45.6485, 81.0041) centre (-34.2595, 54.8419) ccw construction
  arc A436 (-45.6485, 81.0041) -> (-45.6335, 78.4447) centre (-1.6604, 79.9828) ccw construction
  arc A437 (-45.6335, 78.4447) -> (-38.7605, 76.5172) centre (-34.5527, 104.7388) ccw construction
  arc A438 (-38.7605, 76.5172) -> (-38.4962, 74.3659) centre (-1.6604, 79.9828) ccw construction
  arc A439 (-38.4962, 74.3659) -> (-44.6983, 70.8322) centre (-27.5829, 48.0017) ccw construction
  arc A440 (-44.6983, 70.8322) -> (-44.0935, 68.3452) centre (-1.6604, 79.9828) ccw construction
  arc A441 (-44.0935, 68.3452) -> (-36.9612, 68.0547) centre (-39.3752, 96.4861) ccw construction
  arc A442 (-36.9612, 68.0547) -> (-36.2079, 66.0223) centre (-1.6604, 79.9828) ccw construction
  arc A443 (-36.2079, 66.0223) -> (-41.428, 61.1536) centre (-19.5088, 42.8856) ccw construction
  arc A444 (-41.428, 61.1536) -> (-40.2659, 58.8732) centre (-1.6604, 79.9828) ccw construction
  arc A445 (-40.2659, 58.8732) -> (-33.2589, 60.2353) centre (-42.1645, 87.3436) ccw construction
  arc A446 (-33.2589, 60.2353) -> (-32.0572, 58.4314) centre (-1.6604, 79.9828) ccw construction
  arc A447 (-32.0572, 58.4314) -> (-36.0137, 52.4901) centre (-10.4725, 39.7694) ccw construction
  arc A448 (-36.0137, 52.4901) -> (-34.3571, 50.5391) centre (-1.6604, 79.9828) ccw construction
  arc A449 (-34.3571, 50.5391) -> (-27.8531, 53.4805) centre (-42.7702, 77.8043) ccw construction
  arc A450 (-27.8531, 53.4805) -> (-26.2678, 52.0024) centre (-1.6604, 79.9828) ccw construction
  arc A451 (-26.2678, 52.0024) -> (-28.7475, 45.3087) centre (-0.9612, 38.8212) ccw construction
  arc A452 (-28.7475, 45.3087) -> (-26.6855, 43.7924) centre (-1.6604, 79.9828) ccw construction
  arc A453 (-26.6855, 43.7924) -> (-21.0352, 48.1544) centre (-41.1597, 68.3824) ccw construction
  arc A454 (-21.0352, 48.1544) -> (-19.1518, 47.0817) centre (-1.6604, 79.9828) ccw construction
  arc A455 (-19.1518, 47.0817) -> (-20.021, 39.9967) centre (8.5125, 40.0919) ccw construction
  arc A456 (-20.021, 39.9967) -> (-17.6649, 38.9967) centre (-1.6604, 79.9828) ccw construction
  arc A457 (-17.6649, 38.9967) -> (-13.1728, 44.5442) centre (-37.4198, 59.5859) ccw construction
  arc A458 (-13.1728, 44.5442) -> (-11.0928, 43.9348) centre (-1.6604, 79.9828) ccw construction
  arc A459 (-11.0928, 43.9348) -> (-10.3046, 36.8403) centre (17.4378, 43.5132) ccw construction
  arc A460 (-10.3046, 36.8403) -> (-7.7815, 36.4106) centre (-1.6604, 79.9828) ccw construction
  arc A461 (-7.7815, 36.4106) -> (-4.6898, 42.8445) centre (-31.752, 51.889) ccw construction
  arc A462 (-4.6898, 42.8445) -> (-2.5253, 42.7312) centre (-1.6604, 79.9828) ccw construction
  arc A463 (-66.9339, 20.4902) -> (66.0259, 23.2504) centre (0, 0) ccw
  arc A464 (40.7849, 94.9294) -> (-44.6893, 93.1551) centre (-1.6604, 79.9828) ccw
  line L4 (-66.9339, 20.4902) -> (-44.6893, 93.1551)
  line L5 (40.7849, 94.9294) -> (66.0259, 23.2504)
  arc A465 (45.501, 96.5902) -> (-49.4703, 94.6186) centre (-1.6604, 79.9828) ccw
  line L6 (45.501, 96.5902) -> (70.742, 24.9111)
  arc A466 (-71.7149, 21.9538) -> (70.742, 24.9111) centre (0, 0) ccw
  line L7 (-71.7149, 21.9538) -> (-49.4703, 94.6186)
  dimension "d0" = 70
  dimension "d1" = 45
  dimension "d2" = 5
  constraints: 8 end point, 8 point on circle, 4 centre point, 4 tangent, 2 coincident, 3 other
  measures "d0" radius of A463
  measures "d1" radius of A464
  measures "d2" radial gap between concentric circles of A463 A466
extrude "Extrusion1" add sketch "Sketch1" along normal blind 10 contours L4 A464 L5 A463 | L6 A466 L7 A465
sketch "Sketch2" plane through (0, 0, 10) normal (0, 0, 1) x (1, 0, 0)
  circle A0 centre (-1.6604, 79.9828) radius 17.5 projected
  circle A1 centre (0, 0) radius 17.5 projected
  arc A2 (45.501, 96.5902) -> (-49.4703, 94.6186) centre (-1.6604, 79.9828) ccw projected
  line L0 (-49.4703, 94.6186) -> (-71.7149, 21.9538) projected
  arc A3 (-71.7149, 21.9538) -> (70.742, 24.9111) centre (0, 0) ccw projected
  line L1 (70.742, 24.9111) -> (45.501, 96.5902) projected
  circle A4 centre (-1.6604, 79.9828) radius 6.75
  dimension "d5" = 13.5
  constraints: 1 centre point, 1 coincident
  measures "d5" diameter of A4
extrude "Extrusion2" add sketch "Sketch2" along normal blind 4 contours A0 | A1 | L1 A3 L0 A2
body "Solid1"
